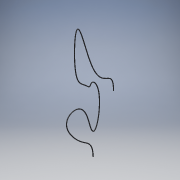
# Autodesk Inventor part: shingeki no kyojin Gas wire
Saved by Autodesk Inventor 2021 (Build 250183000, 183)
## iProperties
Created: 2014-03-28
Part Number: shingeki no kyojin Gas wire
Material: Generic
Document SubType Name: Modeling
Designer: T420s
Density: 1 g/cm^3
Appearance: Default
Author: T420s
Autodesk Inventor part; units mm, degrees
ref_plane "YZ Plane" through (0, 0, 0) normal (1, 0, 0) x (0, 1, 0)
ref_plane "XY Plane" through (0, 0, 0) normal (0, 0, 1) x (1, 0, 0)
sketch "Sketch1" plane through (0, 0, 0) normal (1, 0, 0) x (0, 1, 0)
  line L0 (-70.9946, -17.7837) -> (-34.7656, -17.7837) construction
  line L1 (-34.7656, -17.7837) -> (-13.4102, 7.5496) construction
  line L2 (-13.4102, 7.5496) -> (-13.4102, 25.639) construction
  line L3 (-13.4102, 25.639) -> (93.06, 114.8696) construction
  line L4 (93.06, 114.8696) -> (126.716, 2.6448) construction
  line L5 (126.716, 2.6448) -> (-8.0871, -5.8606) construction
  line L6 (-8.0871, -5.8606) -> (-3.9107, -34.8853) construction
  line L7 (-3.9107, -34.8853) -> (130.0541, -50.2614) construction
  line L8 (130.0541, -50.2614) -> (172.7186, -5.5139) construction
  line L9 (172.7186, -5.5139) -> (130.0541, -11.1672) construction
  line L10 (130.0541, -11.1672) -> (173.0378, 14.4639) construction
  line L11 (173.0378, 14.4639) -> (172.7186, 58.7572) construction
  line L12 (172.7186, 58.7572) -> (520.281, 40.5401) construction
  line L13 (520.281, 40.5401) -> (60.58, -20.3729) construction
  line L14 (60.58, -20.3729) -> (170.1807, -89.0615) construction
  line L15 (170.1807, -89.0615) -> (93.06, -89.0615) construction
  spline S0 degree 4 poles (-70.9946, -17.7837) (-34.7656, -17.7837) (-13.4102, 7.5496) (-13.4102, 25.639) (93.06, 114.8696) (126.716, 2.6448) (-8.0871, -5.8606) (-3.9107, -34.8853) (130.0541, -50.2614) (172.7186, -5.5139) (130.0541, -11.1672) (173.0378, 14.4639) (172.7186, 58.7572) (520.281, 40.5401) (60.58, -20.3729) (170.1807, -89.0615) (93.06, -89.0615) knots 1 1 1 1 1 2 3 4 5 6 7 8 9 10 11 12 13 14 14 14 14 14
  point P0 (0, 0)
  constraints: 2 horizontal, 2 point on line, 3 other
sketch "Sketch2" plane through (0, 0, 0) normal (0, 1, 0) x (-1, 0, 0)
  point P0 (0, 0)
ref_plane "Work Plane1" through (0, -70.9946, -17.7837) normal (0, 1, 0) x (-1, 0, 0)
sketch "Sketch3" plane through (0, -70.9946, -17.7837) normal (0, 1, 0) x (-1, 0, 0)
  circle A0 centre (0, 0) radius 1.4221
  point P0 (0, 17.7837)
  constraints: 1 centre point, 1 coincident
sweep "Sweep2" add profiles "Sketch3" path "Sketch1"
body "Solid2"
